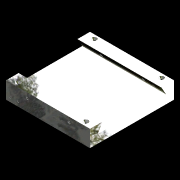
# Autodesk Inventor part: 3d_LM-Welding_Tooling - Upper fixed base
Saved by Autodesk Inventor 2018.3 (Build 223284000, 284)
## iProperties
Created: 2026-01-26
Part Number: 3d_LM-Welding_Tooling - Upper fixed base
Material: Aluminium 6061-T6
Document SubType Name: Modeling
Designer: aca6
Density: 2.7 g/cm^3
Appearance: N/A - Machined Aluminium
Manufacturer-1: {"Name": "Hanstar Technologies Co., Ltd", "PartNumber": "3d_Welding_Tooling - Upper fixed base", "Link": ""}
Manufacturer-2: {"Name": "SHENZHEN JINYIHE PROTOTYPE TECHNOLOGIES CO., LTD", "PartNumber": "3d_Welding_Tooling - Upper fixed base", "Link": ""}
Manufacturer-3: {"Name": "Shenzhen city Xavier Precision Co., Ltd.", "PartNumber": "3d_Welding_Tooling - Upper fixed base", "Link": ""}
Manufacturer-4: {"Name": "", "PartNumber": "", "Link": ""}
Manufacturer-5: {"Name": "", "PartNumber": "", "Link": ""}
Provider-1: {"Name": "", "PartNumber": "", "Link": ""}
Provider-2: {"Name": "", "PartNumber": "", "Link": ""}
Provider-3: {"Name": "", "PartNumber": "", "Link": ""}
Provider-4: {"Name": "", "PartNumber": "", "Link": ""}
Provider-5: {"Name": "", "PartNumber": "", "Link": ""}
Author: aca6
Comments: DIN-ISO-2768-fH
Autodesk Inventor part; units mm, degrees
ref_plane "YZ Plane" through (0, 0, 0) normal (1, 0, 0) x (0, 1, 0)
ref_plane "XZ Plane" through (0, 0, 0) normal (0, 1, 0) x (-1, 0, 0)
ref_plane "XY Plane" through (0, 0, 0) normal (0, 0, 1) x (1, 0, 0)
sketch "Sketch1" plane through (0, 0, 0) normal (0, 0, 1) x (1, 0, 0)
  line L0 (-50, 50) -> (50, 50)
  line L1 (50, 50) -> (50, -50)
  line L2 (50, -50) -> (-50, -50)
  line L3 (-50, -50) -> (-50, 50)
  line L4 (0, 0) -> (0, 10.7298) construction
  line L5 (0, 0) -> (15.4092, 0) construction
  dimension "d0" = 100
  dimension "d1" = 100
  constraints: 12 end point, 3 horizontal, 2 parallel, 2 vertical, 1 perpendicular, 4 other
  measures "d0" distance of L0.end L1.end
  measures "d1" distance of L0.start L0.end
extrude "Extrusion1" add sketch "Sketch1" along normal blind 20
sketch "Sketch2" plane through (50, -50, 0) normal (1, 0, 0) x (0, 0, -1)
  line L0 (-20, 100) -> (-20, 0)
  line L1 (-20, 15) -> (-10, 9.2265)
  line L2 (-10, 9.2265) -> (-10, 90.7735)
  line L3 (-10, 90.7735) -> (-20, 85)
  line L4 (0, 0) -> (-20, 0) projected
  line L5 (0, 100) -> (-20, 100) projected
  point P0 (0, 50)
  dimension "d4" = 60
  dimension "d5" = 60
  dimension "d6" = 10
  dimension "d9" = 15
  dimension "d10" = 15
  constraints: 8 end point, 2 point on line, 1 parallel
  measures "d4" angle of L2 L1
  measures "d5" angle of L2 L3
  measures "d6" distance between parallel lines of L0 L2
  measures "d9" distance from line of L4 L1.start
  measures "d10" distance from line of L5 L3.end
extrude "Extrusion2" cut sketch "Sketch2" against normal blind 115.5
sketch "Sketch4" plane through (0, 0, 20) normal (0, 0, 1) x (1, 0, 0)
  line L0 (-50, -50) -> (50, -50) projected
  line L1 (-50, -35) -> (-50, -50) projected
  line L2 (50, -50) -> (50, -35) projected
  line L3 (-50, 50) -> (-50, 35) projected
  line L4 (50, 50) -> (-50, 50) projected
  line L5 (50, 35) -> (50, 50) projected
  circle A0 centre (-40, -45) radius 3
  circle A1 centre (40, -45) radius 3
  circle A2 centre (-40, 45) radius 3
  circle A3 centre (40, 45) radius 3
  point P0 (0, 0)
  dimension "d28" = 5
  dimension "d29" = 10
  dimension "d30" = 5
  dimension "d31" = 10
  dimension "d32" = 10
  dimension "d33" = 5
  dimension "d34" = 10
  dimension "d35" = 5
  dimension "d36" = 6
  dimension "d37" = 6
  dimension "d38" = 6
  dimension "d39" = 6
  constraints: 4 centre point, 4 coincident
  measures "d28" distance from line of L0 point (-40, -45)
  measures "d29" distance from line of L1 point (-40, -45)
  measures "d30" distance from line of L0 point (40, -45)
  measures "d31" distance from line of L2 point (40, -45)
  measures "d32" distance from line of L3 point (-40, 45)
  measures "d33" distance from line of L4 point (-40, 45)
  measures "d34" distance from line of L5 point (40, 45)
  measures "d35" distance from line of L4 point (40, 45)
  measures "d36" diameter of A0
  measures "d37" diameter of A1
  measures "d38" diameter of A2
  measures "d39" diameter of A3
extrude "Extrusion3" cut sketch "Sketch4" against normal blind 0.3
sketch "Sketch5" plane through (-40, 45, 19.7) normal (0, 0, 1) x (1, 0, 0)
  circle A0 centre (0, -90) radius 3 projected
  circle A1 centre (0, 0) radius 3 projected
  circle A2 centre (80, 0) radius 3 projected
  circle A3 centre (80, -90) radius 3 projected
  point P0 (40, -45)
  constraints: 4 coincident
hole "Hole2" at (-40, -45, 19.7) at (-40, 45, 19.7) at (40, 45, 19.7) at (40, -45, 19.7) direction (0, 0, -1) diameter 2.459 end through all countersink diameter 6 countersink angle 90 thread size "M3x0.5" class "6H" standard "ISO Metric profile"
sketch "Sketch6" plane through (-50, -50, 0) normal (0, -1, 0) x (1, 0, 0)
  line L0 (0, 20) -> (100, 20) projected
  line L1 (100, 0) -> (0, 0) projected
  line L2 (100, 0) -> (100, 20) projected
  line L3 (0, 0) -> (0, 20) projected
  point P0 (50, 0)
  point P1 (75, 14)
  point P2 (50, 0)
  point P3 (25, 14)
  dimension "d49" = 6
  dimension "d57" = 25
  dimension "d65" = 25
  constraints: 1 horizontal alignment, 1 midpoint
  measures "d49" distance from line of L0 point (75, 14)
  measures "d57" distance from line of L2 point (75, 14)
  measures "d65" distance from line of L3 point (25, 14)
hole "Hole3" at (25, -50, 14) at (-25, -50, 14) direction (0, 1, 0) diameter 3.242 end through all thread size "M4x0.7" class "6H" standard "ISO Metric profile"
sketch "Sketch7" plane through (-50, -50, 0) normal (0, -1, 0) x (1, 0, 0)
  circle A0 centre (14, 5) radius 1.6 projected
  circle A1 centre (5, 5) radius 1.6 projected
  point P0 (50, 0)
  constraints: 2 coincident
hole "Hole4" at (-45, -50, 5) at (-36, -50, 5) direction (0, 1, 0) diameter 2.459 depth 9 tip angle 118 thread size "M3x0.5" class "6H" standard "ISO Metric profile"
body "Solid1"
